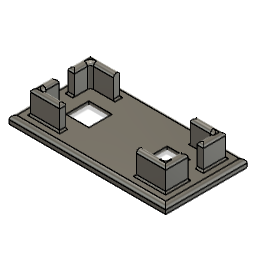
JIG (Autodesk Fusion 360 design; units mm, degrees)
Autodesk Fusion 360 part; units mm, degrees
note: some values were not read from the file. Chosen so that the rebuilt part matches the saved one: which face or edge a step refers to.
sketch "Sketch1" plane through (0, 0, 0) normal (0, 1, 0) x (1, 0, 0)
  line L0 (51, 26.5) -> (-51, 26.5)
  line L1 (-51, 26.5) -> (-51, -26.5)
  line L2 (-51, -26.5) -> (51, -26.5)
  line L3 (51, -26.5) -> (51, 26.5)
  line L4 (51, 26.5) -> (-51, -26.5) construction
  line L5 (-51, 26.5) -> (51, -26.5) construction
  dimension "d1" = 102
  dimension "d2" = 53
  constraint horizontal L0
  constraint perpendicular L0 L1
  constraint parallel L0 L2
  constraint parallel L1 L3
  constraint coincident L4 origin
  constraint coincident L5 origin
  measures "d1" distance of L1.end L2.end
  measures "d2" distance of L0.end L1.end
extrude "Extrude1" add sketch "Sketch1" along normal blind 7
sketch "Sketch2" plane through (0, 7, 0) normal (0, 1, 0) x (-1, 0, 0)
  line L0 (-51, 26.5) -> (-51, -26.5)
  line L1 (-51, -26.5) -> (51, -26.5)
  line L2 (51, -26.5) -> (51, 26.5)
  line L3 (51, 26.5) -> (-51, 26.5)
  line L4 (-44, -19.5) -> (44, -19.5)
  line L5 (44, -19.5) -> (44, 19.5)
  line L6 (44, 19.5) -> (-44, 19.5)
  line L7 (-44, 19.5) -> (-44, -19.5)
  line L8 (-44, -19.5) -> (44, 19.5) construction
  line L9 (44, -19.5) -> (-44, 19.5) construction
  line L10 (-40, -15.5) -> (40, -15.5)
  line L11 (40, -15.5) -> (40, 15.5)
  line L12 (40, 15.5) -> (-40, 15.5)
  line L13 (-40, 15.5) -> (-40, -15.5)
  line L14 (-40, -15.5) -> (40, 15.5) construction
  line L15 (40, -15.5) -> (-40, 15.5) construction
  dimension "d5" = 88
  dimension "d6" = 39
  dimension "d7" = 80
  dimension "d8" = 31
  constraint horizontal L4
  constraint perpendicular L4 L5
  constraint parallel L4 L6
  constraint parallel L5 L7
  constraint coincident L8 origin
  constraint coincident L9 origin
  constraint horizontal L10
  constraint perpendicular L10 L11
  constraint parallel L10 L12
  constraint parallel L11 L13
  constraint coincident L14 origin
  constraint coincident L15 origin
  measures "d5" distance of L5.end L6.end
  measures "d6" distance of L4.end L5.end
  measures "d7" distance of L11.end L12.end
  measures "d8" distance of L10.end L11.end
extrude "Extrude2" add sketch "Sketch2" along normal blind 15 contours L4 L5 L6 L7
fillet "Fillet1" radius 2 4 edges at (-40, 14.5, -15.5) (-40, 14.5, 15.5) (40, 14.5, 15.5) (40, 14.5, -15.5)
sketch "Sketch3" plane through (0, 0, 0) normal (0, -1, 0) x (1, 0, 0)
  line L0 (51, -26.5) -> (51, 26.5)
  line L1 (51, 26.5) -> (-51, 26.5)
  line L2 (-51, 26.5) -> (-51, -26.5)
  line L3 (-51, -26.5) -> (51, -26.5)
  line L4 (-51, 26.5) -> (0, -26.5) construction
  line L5 (51, 26.5) -> (0, -26.5) construction
  line L6 (0, 26.5) -> (51, -26.5) construction
  line L7 (-51, -26.5) -> (0, 26.5) construction
  line L8 (-18, -7.5) -> (-33, -7.5)
  line L9 (-33, -7.5) -> (-33, 7.5)
  line L10 (-33, 7.5) -> (-18, 7.5)
  line L11 (-18, 7.5) -> (-18, -7.5)
  line L12 (-18, -7.5) -> (-33, 7.5) construction
  line L13 (-33, -7.5) -> (-18, 7.5) construction
  line L14 (33, 7.5) -> (18, 7.5)
  line L15 (18, 7.5) -> (18, -7.5)
  line L16 (18, -7.5) -> (33, -7.5)
  line L17 (33, -7.5) -> (33, 7.5)
  line L18 (33, 7.5) -> (18, -7.5) construction
  line L19 (18, 7.5) -> (33, -7.5) construction
  point P0 (-25.5, 0)
  point P1 (25.5, 0)
  dimension "d13" = 15
  dimension "d14" = 15
  dimension "d15" = 15
  dimension "d16" = 15
  constraint coincident L1.end L2.start
  constraint midpoint L3 L4.end
  constraint coincident L0.end L1.start
  constraint midpoint L1 L6.start
  constraint coincident L0.start L3.end
  constraint coincident L2.end L3.start
  constraint horizontal L8
  constraint perpendicular L8 L9
  constraint parallel L8 L10
  constraint parallel L9 L11
  constraint coincident L12 P0
  constraint coincident L13 P0
  constraint midpoint L7 P0
  constraint horizontal L14
  constraint perpendicular L14 L15
  constraint parallel L14 L16
  constraint parallel L15 L17
  constraint coincident L18 P1
  constraint coincident L19 P1
  constraint midpoint L6 P1
  measures "d13" distance of L9.end L10.end
  measures "d14" distance of L8.end L9.end
  measures "d15" distance of L15.end L16.end
  measures "d16" distance of L14.end L15.end
extrude "Extrude3" cut sketch "Sketch3" against normal blind 7 contours L8 L9 L10 L11 | L14 L15 L16 L17
extrude "Extrude4" cut 1 faces at (-6, 0, 20.1667) along direction (0, 1, 0) blind 2
move_body "Move1" bodies 1 to x (1, 0, 0) y (0, 1, 0) z (0, 0, 1) at (0, -2, 0)
fillet "Fillet4" radius 2.5 4 edges at (51, 5, 0) (0, 5, -26.5) (-51, 5, 0) (0, 5, 26.5)
fillet "Fillet5" radius 5 8 edges at (18, 0, 0) (25.5, 0, -7.5) (33, 0, 0) (25.5, 0, 7.5) (-25.5, 0, 7.5) (-33, 0, 0) (-25.5, 0, -7.5) (-18, 0, 0)
sketch "Sketch4" plane through (0, 20, 0) normal (0, 1, 0) x (-1, 0, 0)
  line L0 (-40, -13.5) -> (-40, 13.5)
  arc A0 (-38, 15.5) -> (-40, 13.5) centre (-38, 13.5) ccw
  line L1 (-38, 15.5) -> (38, 15.5)
  arc A1 (40, 13.5) -> (38, 15.5) centre (38, 13.5) ccw
  line L2 (40, 13.5) -> (40, -13.5)
  arc A2 (38, -15.5) -> (40, -13.5) centre (38, -13.5) ccw
  line L3 (38, -15.5) -> (-38, -15.5)
  arc A3 (-40, -13.5) -> (-38, -15.5) centre (-38, -13.5) ccw
  line L4 (-44, 19.5) -> (-44, -19.5)
  line L5 (-44, -19.5) -> (44, -19.5)
  line L6 (44, -19.5) -> (44, 19.5)
  line L7 (44, 19.5) -> (-44, 19.5)
  line L8 (25, -15.5) -> (25, -19.5)
  line L9 (-25, -15.5) -> (-25, -19.5)
  line L10 (25, 15.5) -> (25, 19.5)
  line L11 (-25, 15.5) -> (-25, 19.5)
  line L12 (25, -19.5) -> (-25, -19.5)
  line L13 (-25, -15.5) -> (25, -15.5)
  line L14 (25, 15.5) -> (-25, 15.5)
  line L15 (-25, 19.5) -> (25, 19.5)
  dimension "d29" = 13
  dimension "d30" = 13
  constraint coincident L5 L8.end
  constraint perpendicular L5 L8
  constraint coincident L5 L9.end
  constraint perpendicular L5 L9
  constraint coincident L1 L11.start
  constraint coincident L1 L10.start
  constraint coincident L7 L10.end
  constraint perpendicular L7 L10
  constraint coincident L7 L11.end
  constraint perpendicular L7 L11
  constraint perpendicular L9 L13
  constraint perpendicular L11 L14
  measures "d29" distance of A2.start L8.start
  measures "d30" distance of L3.end L9.start
extrude "Extrude5" cut sketch "Sketch4" against normal blind 15 contours L3 L5 L8 L9 L12 L13 | L1 L7 L10 L11 L14 L15
sketch "Sketch5" plane through (0, 20, 0) normal (0, 1, 0) x (-1, 0, 0)
  line L0 (25, -15.5) -> (25, -19.5)
  line L1 (25, -19.5) -> (44, -19.5)
  line L2 (44, -19.5) -> (44, 19.5)
  line L3 (44, 19.5) -> (25, 19.5)
  line L4 (25, 19.5) -> (25, 15.5)
  line L5 (25, 15.5) -> (38, 15.5)
  arc A0 (40, 13.5) -> (38, 15.5) centre (38, 13.5) ccw
  line L6 (40, 13.5) -> (40, -13.5)
  arc A1 (38, -15.5) -> (40, -13.5) centre (38, -13.5) ccw
  line L7 (38, -15.5) -> (25, -15.5)
  line L8 (44, 0) -> (44, -5)
  line L9 (44, -5) -> (40, -5)
  line L10 (40, -5) -> (40, 5)
  line L11 (40, 5) -> (44, 5)
  line L12 (44, -5) -> (44, 5)
  dimension "d33" = 5
  dimension "d34" = 10
  dimension "d35" = 4
  constraint midpoint L2 L8.start
  constraint parallel L2 L8
  constraint coincident L6 L9.end
  constraint perpendicular L6 L9
  constraint coincident L6 L10.end
  constraint perpendicular L2 L11
  measures "d33" distance of L8.start L8.end
  measures "d34" distance of L9.end L10.end
  measures "d35" distance of L10.end L11.end
extrude "Extrude6" cut sketch "Sketch5" against normal blind 15 contours L2 L6 L8 L9 L10 L11 L12
sketch "Sketch6" plane through (0, 20, 0) normal (0, 1, 0) x (-1, 0, 0)
  line L0 (-25, -19.5) -> (-25, -15.5)
  line L1 (-25, -15.5) -> (-38, -15.5)
  arc A0 (-40, -13.5) -> (-38, -15.5) centre (-38, -13.5) ccw
  line L2 (-40, -13.5) -> (-40, 13.5)
  arc A1 (-38, 15.5) -> (-40, 13.5) centre (-38, 13.5) ccw
  line L3 (-38, 15.5) -> (-25, 15.5)
  line L4 (-25, 15.5) -> (-25, 19.5)
  line L5 (-25, 19.5) -> (-44, 19.5)
  line L6 (-44, 19.5) -> (-44, -19.5)
  line L7 (-44, -19.5) -> (-25, -19.5)
  line L8 (-40, 0) -> (-40, -5)
  line L9 (-40, 0) -> (-40, 5)
  line L10 (-40, -5) -> (-44, -5)
  line L11 (-44, -5) -> (-44, 5)
  line L12 (-44, 5) -> (-40, 5)
  line L13 (-40, 5) -> (-40, -5)
  dimension "d38" = 5
  dimension "d39" = 5
  dimension "d40" = 4
  dimension "d41" = 10
  constraint midpoint L2 L8.start
  constraint parallel L2 L8
  constraint coincident L2 L9.end
  constraint horizontal L10
  constraint vertical L11
  constraint horizontal L12
  constraint vertical L13
  measures "d38" distance of L8.start L8.end
  measures "d39" distance of L8.start L9.end
  measures "d40" distance of L8.end L10.end
  measures "d41" distance of L8.end L9.end
extrude "Extrude7" cut sketch "Sketch6" against normal blind 15 contours L2 L6 L8 L9 L10 L11 L12 L13
fillet "Fillet6" radius 2 26 edges at (40, 20, 9.25) (40, 20, -9.25) (39.4142, 20, -14.9142) (31.5, 20, -15.5) (25, 20, -17.5) (34.5, 20, -19.5) (44, 20, 12.25) (44, 20, -12.25) (34.5, 20, 19.5) (31.5, 20, 15.5) (39.4142, 20, 14.9142) (-31.5, 20, 15.5) (-25, 20, 17.5) (-34.5, 20, 19.5) (-44, 20, 12.25) (-42, 20, 5) (-40, 20, 9.25) (-39.4142, 20, 14.9142) (-44, 20, -12.25) (-34.5, 20, -19.5) (-31.5, 20, -15.5) (-39.4142, 20, -14.9142) (-40, 20, -9.25) (-42, 20, -5) (42, 20, 5) (42, 20, -5)
fillet "Fillet7" radius 1 6 edges at (44, 5, 12.25) (34.5, 5, 19.5) (44, 5, -12.25) (34.5, 5, -19.5) (-34.5, 5, -19.5) (-44, 5, -12.25)
fillet "Fillet8" radius 1 2 edges at (-34.5, 5, 19.5) (-44, 5, 12.25)
fillet "Fillet9" radius 1 4 edges at (25, 5, -18) (25, 5, 18) (-25, 5, -18) (-25, 5, 18)
fillet "Fillet10" radius 1 4 edges at (42.5, 5, -5) (-42.5, 5, -5) (42.5, 5, 5) (-42.5, 5, 5)
fillet "Fillet2" [suppressed]
fillet "Fillet3" [suppressed]
